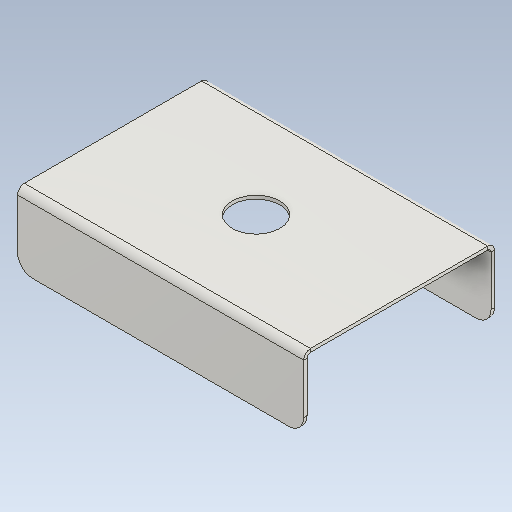
# Autodesk Inventor part: guarda_conector_ceramico
Saved by Autodesk Inventor 2021 (Build 250183000, 183)
## iProperties
Created: 2021-04-19
Part Number: guarda_conector_ceramico
Material: Acero AISI 1006 85 LC
Document SubType Name: Chapa
Designer: Leonardo Fabio Mercado Benítez
Density: 7.872 g/cm^3
Sheet Metal Rule: Por defecto_mm
Appearance: Acero
Mass: 5.67519 g
Surface Area: 32.8455 cm^2
Volume: 0.720934 cm^3
Author: Leonardo Fabio Mercado Benítez
Autodesk Inventor part; units mm, degrees
ref_plane "YZ Plane" through (0, 0, 0) normal (1, 0, 0) x (0, 1, 0)
ref_plane "XZ Plane" through (0, 0, 0) normal (0, 1, 0) x (-1, 0, 0)
ref_plane "XY Plane" through (0, 0, 0) normal (0, 0, 1) x (1, 0, 0)
sketch "Boceto1" plane through (0, 0, 0) normal (0, 1, 0) x (-1, 0, 0)
  line L0 (19.05, -12.7) -> (-19.05, -12.7)
  line L1 (-19.05, -12.7) -> (-19.05, 12.7)
  line L2 (-19.05, 12.7) -> (19.05, 12.7)
  line L3 (19.05, 12.7) -> (19.05, -12.7)
  line L4 (19.05, -12.7) -> (-19.05, 12.7) construction
  line L5 (-19.05, -12.7) -> (19.05, 12.7) construction
  point P0 (0, 0)
  dimension "d0" = 38.1
  dimension "d1" = 25.4
  measures "d0" distance of L1.end L2.end
  measures "d1" distance of L0.end L1.end
extrude "Placa1" add sketch "Boceto1" along normal blind 0.45
sketch "Boceto2" plane through (-19.05, 0.45, 12.25) normal (0, 0, 1) x (1, 0, 0)
  line L0 (38.1, 0) -> (0, 0)
  line L1 (0, 0) -> (0, -9.525)
  line L2 (0, -9.525) -> (38.1, -9.525)
  line L3 (38.1, -9.525) -> (38.1, 0)
  constraints: 6 end point, 1 horizontal, 1 perpendicular, 1 vertical
edge flange "Pestaña1" height 9.525 angle 90 thickness 0.45 bend radius 0.45 thickness toward (0, 0, 1) relief straight relief width 0.45 relief depth 0.225 corner gap 0.45 corner form 0 edges at (0, 0, 12.7) (0, 0, -12.7) wall of the first edge with corners at (19.05, 0.45, 12.25) (-19.05, 0.45, 12.25) (-19.05, -9.075, 12.25) (19.05, -9.075, 12.25)
bend "Doblez1"
corner "Esquina1"
fillet "Empalme1" radius 2 4 edges at (19.05, -9.075, 12.475) (19.05, -9.075, -12.475) (-19.05, -9.075, 12.475) (-19.05, -9.075, -12.475)
sketch "Boceto3" plane through (0, 0.45, 0) normal (0, 1, 0) x (1, 0, 0)
  circle A0 centre (0, 0) radius 3.175
  dimension "d14" = 6.35
  constraints: 1 centre point, 1 coincident
  measures "d14" diameter of A0
extrude "Cortar1" cut sketch "Boceto3" against normal blind 0.45
equation "\"d15\" = Grosor"
equation "\"d2\" = Grosor"
equation "\"d3\" = Anchura_desahogo_plegado"
equation "\"d4\" = Profundidad_desahogo_plegado"
equation "\"d5\" = Remanente_mínimo"
equation "\"d6\" = Radiodetransición"
equation "\"d9\" = Radio_pliegue"
equation "\"d10\" = Tamaño_destalonado"
equation "\"d11\" = TamañoSeparación"
equation "\"d12\" = Tamaño_de_radio_de_Jacobi"
equation "\"Radio_pliegue\" = Grosor"
equation "\"Anchura_desahogo_plegado\" = Grosor"
equation "\"Profundidad_desahogo_plegado\" = 0.5 * Grosor"
equation "\"Tamaño_destalonado\" = 4 * Grosor"
equation "\"Remanente_mínimo\" = 2 * Grosor"
equation "\"Radiodetransición\" = Radio_pliegue"
equation "\"Tamaño_de_radio_de_Jacobi\" = Radio_pliegue"
equation "\"TamañoSeparación\" = Grosor"
equation "\"Grosor\" = 0.45"
